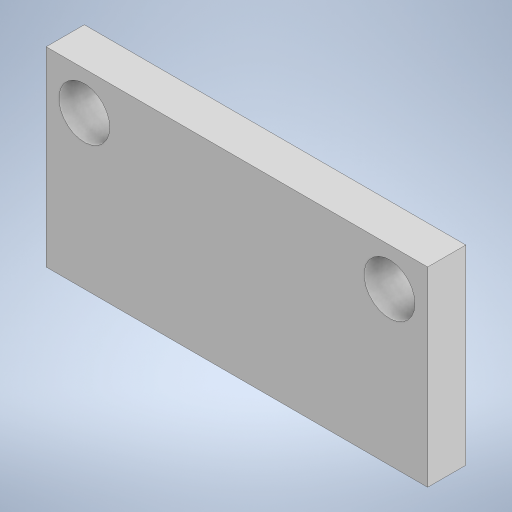
# Autodesk Inventor part: imu_holder
Saved by Autodesk Inventor 2024 (Build 280153000, 153)
## iProperties
Created: 2023-07-30
Part Number: imu_holder
Material: Generic
Document SubType Name: Modeling
Designer: Pintu
Density: 1 g/cm^3
Appearance: Default
Author: Pintu
Autodesk Inventor part; units mm, degrees
ref_plane "YZ Plane" through (0, 0, 0) normal (1, 0, 0) x (0, 1, 0)
ref_plane "XZ Plane" through (0, 0, 0) normal (0, 1, 0) x (-1, 0, 0)
ref_plane "XY Plane" through (0, 0, 0) normal (0, 0, 1) x (1, 0, 0)
sketch "Sketch1" plane through (0, 0, 0) normal (0, 0, 1) x (1, 0, 0)
  line L0 (-15, 7.5) -> (15, 7.5)
  line L1 (15, 7.5) -> (15, -7.5)
  line L2 (15, -7.5) -> (-15, -7.5)
  line L3 (-15, -7.5) -> (-15, 7.5)
  line L4 (-15, 7.5) -> (15, -7.5) construction
  line L5 (15, 7.5) -> (-15, -7.5) construction
  circle A0 centre (-12, 4.5) radius 2
  line L6 (0, -7.5) -> (0, 7.5)
  circle A1 centre (12, 4.5) radius 2
  point P0 (0, 0)
  dimension "d0" = 4
  dimension "d1" = 3
  dimension "d2" = 3
  dimension "d3" = 30
  dimension "d4" = 15
  dimension "d5" = 24
  constraints: 14 end point, 4 midpoint, 2 centre point, 2 parallel, 1 horizontal, 1 perpendicular, 1 symmetric about line, 1 other
  measures "d0" diameter of A0
  measures "d1" distance from line of L0 A0.centre
  measures "d2" distance from line of L3 A0.centre
  measures "d3" distance of L0.start L0.end
  measures "d4" distance of L0.end L1.end
  measures "d5" distance of A1.centre A0.centre
extrude "Extrusion1" add sketch "Sketch1" along normal blind 3
body "Solid1"
